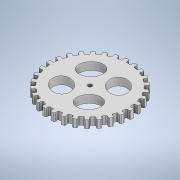
# Autodesk Inventor part: Kolo_zebate
Saved by Autodesk Inventor 2021 (Build 250183000, 183)
## iProperties
Created: 2020-04-11
Part Number: Kolo_zebate
Material: Ogólny
Document SubType Name: Modeling
Designer: dyrag
Density: 1 g/cm^3
Appearance: Domyślna
Author: dyrag
Autodesk Inventor part; units mm, degrees
ref_plane "YZ Plane" through (0, 0, 0) normal (1, 0, 0) x (0, 1, 0)
ref_plane "XZ Plane" through (0, 0, 0) normal (0, 1, 0) x (-1, 0, 0)
ref_plane "XY Plane" through (0, 0, 0) normal (0, 0, 1) x (1, 0, 0)
sketch "Szkic1" plane through (0, 0, 0) normal (0, 1, 0) x (-1, 0, 0)
  circle A0 centre (0, 0) radius 500
  line L0 (550, 0) -> (550, 24.9995)
  line L1 (550, 24.9995) -> (499.3746, 24.9995)
  line L2 (550, 0) -> (550, -25)
  line L3 (550, -25) -> (499.3746, -24.9995)
  line L4 (499.3746, 24.9995) -> (499.3746, -24.9995)
  line L5 (532.7835, 138.8047) -> (483.2644, 128.2791)
  line L6 (543.179, 89.8977) -> (493.6598, 79.3726)
  line L7 (537.9812, 114.3514) -> (532.7835, 138.8047)
  line L8 (537.9812, 114.3514) -> (543.179, 89.8977)
  line L9 (483.2644, 128.2791) -> (493.6598, 79.3726)
  line L10 (492.2818, 246.5434) -> (446.0332, 225.9522)
  line L11 (512.6184, 200.8665) -> (466.3697, 180.2757)
  line L12 (502.45, 223.7052) -> (492.2818, 246.5434)
  line L13 (502.45, 223.7052) -> (512.6184, 200.8665)
  line L14 (446.0332, 225.9522) -> (466.3697, 180.2757)
  line L15 (430.265, 343.5069) -> (389.3082, 313.7501)
  line L16 (459.654, 303.0565) -> (418.6969, 273.3)
  line L17 (444.9593, 323.2819) -> (430.265, 343.5069)
  line L18 (444.9593, 323.2819) -> (459.654, 303.0565)
  line L19 (389.3082, 313.7501) -> (418.6969, 273.3)
  line L20 (349.4436, 425.4576) -> (315.5686, 387.8356)
  line L21 (386.6005, 392.0014) -> (352.7251, 354.3797)
  line L22 (368.0218, 408.7297) -> (349.4436, 425.4576)
  line L23 (368.0218, 408.7297) -> (386.6005, 392.0014)
  line L24 (315.5686, 387.8356) -> (352.7251, 354.3797)
  line L25 (253.3498, 488.8137) -> (228.0371, 444.9709)
  line L26 (296.6506, 463.814) -> (271.3376, 419.9713)
  line L27 (275, 476.314) -> (253.3498, 488.8137)
  line L28 (275, 476.314) -> (296.6506, 463.814)
  line L29 (228.0371, 444.9709) -> (271.3376, 419.9713)
  line L30 (146.1834, 530.8064) -> (130.5393, 482.6588)
  line L31 (193.7358, 515.3557) -> (178.0912, 467.2082)
  line L32 (169.9593, 523.0811) -> (146.1834, 530.8064)
  line L33 (169.9593, 523.0811) -> (193.7358, 515.3557)
  line L34 (130.5393, 482.6588) -> (178.0912, 467.2082)
  line L35 (32.6281, 549.6002) -> (27.3363, 499.2522)
  line L36 (82.3537, 544.3738) -> (77.0615, 494.0258)
  line L37 (57.4907, 546.987) -> (32.6281, 549.6002)
  line L38 (57.4907, 546.987) -> (82.3537, 544.3738)
  line L39 (27.3363, 499.2522) -> (77.0615, 494.0258)
  line L40 (-82.3533, 544.3739) -> (-77.0615, 494.0258)
  line L41 (-32.6276, 549.6003) -> (-27.3363, 499.2522)
  line L42 (-57.4907, 546.987) -> (-82.3533, 544.3739)
  line L43 (-57.4907, 546.987) -> (-32.6276, 549.6003)
  line L44 (-77.0615, 494.0258) -> (-27.3363, 499.2522)
  line L45 (-193.7353, 515.3558) -> (-178.0912, 467.2082)
  line L46 (-146.1829, 530.8065) -> (-130.5393, 482.6588)
  line L47 (-169.9593, 523.0811) -> (-193.7353, 515.3558)
  line L48 (-169.9593, 523.0811) -> (-146.1829, 530.8065)
  line L49 (-178.0912, 467.2082) -> (-130.5393, 482.6588)
  line L50 (-296.6502, 463.8142) -> (-271.3376, 419.9713)
  line L51 (-253.3494, 488.814) -> (-228.0371, 444.9709)
  line L52 (-275, 476.314) -> (-296.6502, 463.8142)
  line L53 (-275, 476.314) -> (-253.3494, 488.814)
  line L54 (-271.3376, 419.9713) -> (-228.0371, 444.9709)
  line L55 (-386.6001, 392.0017) -> (-352.7251, 354.3797)
  line L56 (-349.4432, 425.4579) -> (-315.5686, 387.8356)
  line L57 (-368.0218, 408.7297) -> (-386.6001, 392.0017)
  line L58 (-368.0218, 408.7297) -> (-349.4432, 425.4579)
  line L59 (-352.7251, 354.3797) -> (-315.5686, 387.8356)
  line L60 (-459.6537, 303.0568) -> (-418.6969, 273.3)
  line L61 (-430.2647, 343.5073) -> (-389.3082, 313.7501)
  line L62 (-444.9593, 323.2819) -> (-459.6537, 303.0568)
  line L63 (-444.9593, 323.2819) -> (-430.2647, 343.5073)
  line L64 (-418.6969, 273.3) -> (-389.3082, 313.7501)
  line L65 (-512.6182, 200.8669) -> (-466.3697, 180.2757)
  line L66 (-492.2816, 246.5438) -> (-446.0332, 225.9522)
  line L67 (-502.45, 223.7052) -> (-512.6182, 200.8669)
  line L68 (-502.45, 223.7052) -> (-492.2816, 246.5438)
  line L69 (-466.3697, 180.2757) -> (-446.0332, 225.9522)
  line L70 (-543.1789, 89.8982) -> (-493.6598, 79.3726)
  line L71 (-532.7834, 138.8051) -> (-483.2644, 128.2791)
  line L72 (-537.9812, 114.3514) -> (-543.1789, 89.8982)
  line L73 (-537.9812, 114.3514) -> (-532.7834, 138.8051)
  line L74 (-493.6598, 79.3726) -> (-483.2644, 128.2791)
  line L75 (-550, -24.9995) -> (-499.3746, -24.9995)
  line L76 (-550, 25) -> (-499.3746, 24.9995)
  line L77 (-550, 0) -> (-550, -24.9995)
  line L78 (-550, 0) -> (-550, 25)
  line L79 (-499.3746, -24.9995) -> (-499.3746, 24.9995)
  line L80 (-532.7835, -138.8047) -> (-483.2644, -128.2791)
  line L81 (-543.179, -89.8977) -> (-493.6598, -79.3726)
  line L82 (-537.9812, -114.3514) -> (-532.7835, -138.8047)
  line L83 (-537.9812, -114.3514) -> (-543.179, -89.8977)
  line L84 (-483.2644, -128.2791) -> (-493.6598, -79.3726)
  line L85 (-492.2818, -246.5434) -> (-446.0332, -225.9522)
  line L86 (-512.6184, -200.8665) -> (-466.3697, -180.2757)
  line L87 (-502.45, -223.7052) -> (-492.2818, -246.5434)
  line L88 (-502.45, -223.7052) -> (-512.6184, -200.8665)
  line L89 (-446.0332, -225.9522) -> (-466.3697, -180.2757)
  line L90 (-430.265, -343.5069) -> (-389.3082, -313.7501)
  line L91 (-459.654, -303.0565) -> (-418.6969, -273.3)
  line L92 (-444.9593, -323.2819) -> (-430.265, -343.5069)
  line L93 (-444.9593, -323.2819) -> (-459.654, -303.0565)
  line L94 (-389.3082, -313.7501) -> (-418.6969, -273.3)
  line L95 (-349.4436, -425.4576) -> (-315.5686, -387.8356)
  line L96 (-386.6005, -392.0014) -> (-352.7251, -354.3797)
  line L97 (-368.0218, -408.7297) -> (-349.4436, -425.4576)
  line L98 (-368.0218, -408.7297) -> (-386.6005, -392.0014)
  line L99 (-315.5686, -387.8356) -> (-352.7251, -354.3797)
  line L100 (-253.3498, -488.8137) -> (-228.0371, -444.9709)
  line L101 (-296.6506, -463.814) -> (-271.3376, -419.9713)
  line L102 (-275, -476.314) -> (-253.3498, -488.8137)
  line L103 (-275, -476.314) -> (-296.6506, -463.814)
  line L104 (-228.0371, -444.9709) -> (-271.3376, -419.9713)
  line L105 (-146.1834, -530.8064) -> (-130.5393, -482.6588)
  line L106 (-193.7358, -515.3557) -> (-178.0912, -467.2082)
  line L107 (-169.9593, -523.0811) -> (-146.1834, -530.8064)
  line L108 (-169.9593, -523.0811) -> (-193.7358, -515.3557)
  line L109 (-130.5393, -482.6588) -> (-178.0912, -467.2082)
  line L110 (-32.6281, -549.6002) -> (-27.3363, -499.2522)
  line L111 (-82.3537, -544.3738) -> (-77.0615, -494.0258)
  line L112 (-57.4907, -546.987) -> (-32.6281, -549.6002)
  line L113 (-57.4907, -546.987) -> (-82.3537, -544.3738)
  line L114 (-27.3363, -499.2522) -> (-77.0615, -494.0258)
  line L115 (82.3533, -544.3739) -> (77.0615, -494.0258)
  line L116 (32.6276, -549.6003) -> (27.3363, -499.2522)
  line L117 (57.4907, -546.987) -> (82.3533, -544.3739)
  line L118 (57.4907, -546.987) -> (32.6276, -549.6003)
  line L119 (77.0615, -494.0258) -> (27.3363, -499.2522)
  line L120 (193.7353, -515.3558) -> (178.0912, -467.2082)
  line L121 (146.1829, -530.8065) -> (130.5393, -482.6588)
  line L122 (169.9593, -523.0811) -> (193.7353, -515.3558)
  line L123 (169.9593, -523.0811) -> (146.1829, -530.8065)
  line L124 (178.0912, -467.2082) -> (130.5393, -482.6588)
  line L125 (296.6502, -463.8142) -> (271.3376, -419.9713)
  line L126 (253.3494, -488.814) -> (228.0371, -444.9709)
  line L127 (275, -476.314) -> (296.6502, -463.8142)
  line L128 (275, -476.314) -> (253.3494, -488.814)
  line L129 (271.3376, -419.9713) -> (228.0371, -444.9709)
  line L130 (386.6001, -392.0017) -> (352.7251, -354.3797)
  line L131 (349.4432, -425.4579) -> (315.5686, -387.8356)
  line L132 (368.0218, -408.7297) -> (386.6001, -392.0017)
  line L133 (368.0218, -408.7297) -> (349.4432, -425.4579)
  line L134 (352.7251, -354.3797) -> (315.5686, -387.8356)
  line L135 (459.6537, -303.0568) -> (418.6969, -273.3)
  line L136 (430.2647, -343.5073) -> (389.3082, -313.7501)
  line L137 (444.9593, -323.2819) -> (459.6537, -303.0568)
  line L138 (444.9593, -323.2819) -> (430.2647, -343.5073)
  line L139 (418.6969, -273.3) -> (389.3082, -313.7501)
  line L140 (512.6182, -200.8669) -> (466.3697, -180.2757)
  line L141 (492.2816, -246.5438) -> (446.0332, -225.9522)
  line L142 (502.45, -223.7052) -> (512.6182, -200.8669)
  line L143 (502.45, -223.7052) -> (492.2816, -246.5438)
  line L144 (466.3697, -180.2757) -> (446.0332, -225.9522)
  line L145 (543.1789, -89.8982) -> (493.6598, -79.3726)
  line L146 (532.7834, -138.8051) -> (483.2644, -128.2791)
  line L147 (537.9812, -114.3514) -> (543.1789, -89.8982)
  line L148 (537.9812, -114.3514) -> (532.7834, -138.8051)
  line L149 (493.6598, -79.3726) -> (483.2644, -128.2791)
  dimension "d1" = 1000
  dimension "d3" = 25
  dimension "d6" = 360
  constraints: 300 end point, 30 point on line, 1 perpendicular, 1 vertical, 336 other
  measures "d3" distance of L0.start L2.end
extrude "Wyciągnięcie proste1" add sketch "Szkic1" along normal blind 100
sketch "Szkic2" plane through (0, 0, 0) normal (0, 1, 0) x (-1, 0, 0)
  point P0 (0, 0)
hole "Otwór1" at (0, 0, 0) direction (0, 1, 0) diameter 50 end through all
sketch "Szkic3" plane through (0, 0, 0) normal (0, 1, 0) x (-1, 0, 0)
  ellipse E0 centre (193.4546, 178.9091) end of major axis (84.3637, 276.3637) minor radius 121.2263
  ellipse E1 centre (-178.9091, 193.4546) end of major axis (-276.3637, 84.3637) minor radius 121.2263
  ellipse E2 centre (-193.4546, -178.9091) end of major axis (-84.3637, -276.3637) minor radius 121.2263
  ellipse E3 centre (178.9091, -193.4546) end of major axis (276.3637, -84.3637) minor radius 121.2263
  point P0 (0, 0)
  dimension "d19" = 360
  constraints: 2 centre point, 13 other
extrude "Wyciągnięcie proste2" cut sketch "Szkic3" along normal blind 100
fillet "Zaokrąglenie72" radius 10 120 edges at (-271.3376, 50, -419.9713) (-349.4432, 50, -425.4579) (-386.6001, 50, -392.0017) (-430.2647, 50, -343.5073) (-459.6537, 50, -303.0568) (-492.2816, 50, -246.5438) (-466.3697, 50, -180.2757) (-512.6182, 50, -200.8669) (-532.7834, 50, -138.8051) (-483.2644, 50, -128.2791) (-543.1789, 50, -89.8982) (-493.6598, 50, -79.3726) (-499.3746, 50, -24.9995) (-550, 50, -25) (-493.6598, 50, 79.3726) (-499.3746, 50, 24.9995) (-550, 50, 24.9995) (-512.6184, 50, 200.8665) (-466.3697, 50, 180.2757) (-532.7835, 50, 138.8047) (-483.2644, 50, 128.2791) (-296.6502, 50, -463.8142) (-253.3494, 50, -488.814) (-178.0912, 50, -467.2082) (-352.7251, 50, -354.3797) (-418.6969, 50, -273.3) (-446.0332, 50, -225.9522) (-543.179, 50, 89.8977) (-492.2818, 50, 246.5434) (-459.654, 50, 303.0565) (-430.265, 50, 343.5069) (-386.6005, 50, 392.0014) (-349.4436, 50, 425.4576) (-296.6506, 50, 463.814) (-193.7353, 50, -515.3558) (-146.1829, 50, -530.8065) (-82.3533, 50, -544.3739) (-32.6276, 50, -549.6003) (32.6281, 50, -549.6002) (82.3537, 50, -544.3738) (146.1834, 50, -530.8064) (-130.5393, 50, -482.6588) (-77.0615, 50, -494.0258) (-27.3363, 50, -499.2522) (130.5393, 50, -482.6588) (228.0371, 50, -444.9709) (253.3498, 50, -488.8137) (296.6506, 50, -463.814) (271.3376, 50, -419.9713) (315.5686, 50, -387.8356) (349.4436, 50, -425.4576) (386.6005, 50, -392.0014) (352.7251, 50, -354.3797) (430.265, 50, -343.5069) (459.654, 50, -303.0565) (389.3082, 50, -313.7501) (418.6969, 50, -273.3) (446.0332, 50, -225.9522) (492.2818, 50, -246.5434) (512.6184, 50, -200.8665) (466.3697, 50, -180.2757) (532.7835, 50, -138.8047) (483.2644, 50, -128.2791) (493.6598, 50, -79.3726) (543.179, 50, -89.8977) (550, 50, -24.9995) (499.3746, 50, -24.9995) (550, 50, 25) (499.3746, 50, 24.9995) (493.6598, 50, 79.3726) (543.1789, 50, 89.8982) (532.7834, 50, 138.8051) (483.2644, 50, 128.2791) (512.6182, 50, 200.8669) (466.3697, 50, 180.2757) (492.2816, 50, 246.5438) (446.0332, 50, 225.9522) (459.6537, 50, 303.0568) (418.6969, 50, 273.3) (430.2647, 50, 343.5073) (389.3082, 50, 313.7501) (352.7251, 50, 354.3797) (386.6001, 50, 392.0017) (349.4432, 50, 425.4579) (315.5686, 50, 387.8356) (271.3376, 50, 419.9713) (296.6502, 50, 463.8142) (253.3494, 50, 488.814) (228.0371, 50, 444.9709) (178.0912, 50, 467.2082) (193.7353, 50, 515.3558) (146.1829, 50, 530.8065) (130.5393, 50, 482.6588) (77.0615, 50, 494.0258) (82.3533, 50, 544.3739) (32.6276, 50, 549.6003) (27.3363, 50, 499.2522) (-32.6281, 50, 549.6002) (-27.3363, 50, 499.2522) (-82.3537, 50, 544.3738) (-77.0615, 50, 494.0258) (-146.1834, 50, 530.8064) (-193.7358, 50, 515.3557) (-228.0371, 50, 444.9709) (-253.3498, 50, 488.8137) (-315.5686, 50, 387.8356) (-389.3082, 50, 313.7501) (-446.0332, 50, 225.9522) (-178.0912, 50, 467.2082) (-271.3376, 50, 419.9713) (-352.7251, 50, 354.3797) (-418.6969, 50, 273.3) (-389.3082, 50, -313.7501) (-315.5686, 50, -387.8356) (27.3363, 50, -499.2522) (-228.0371, 50, -444.9709) (178.0912, 50, -467.2082) (193.7358, 50, -515.3557) (77.0615, 50, -494.0258) (-130.5393, 50, 482.6588)
